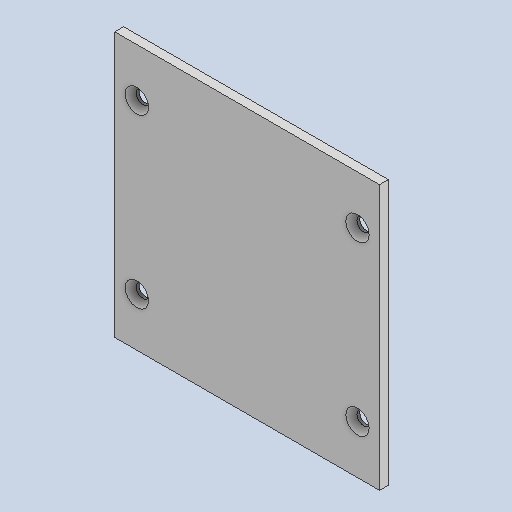
# Autodesk Inventor part: Tapa
Saved by Autodesk Inventor 2023 (Build 270158000, 158)
## iProperties
Created: 2023-04-01
Part Number: Tapa
Material: Genérico
Document SubType Name: Modeling
Designer: sergi
Density: 1 g/cm^3
Appearance: Valor por defecto
Author: sergi
Autodesk Inventor part; units mm, degrees
ref_plane "YZ Plane" through (0, 0, 0) normal (1, 0, 0) x (0, 1, 0)
ref_plane "XZ Plane" through (0, 0, 0) normal (0, 1, 0) x (-1, 0, 0)
ref_plane "XY Plane" through (0, 0, 0) normal (0, 0, 1) x (1, 0, 0)
sketch "Boceto1" plane through (0, 0, 0) normal (0, 0, 1) x (1, 0, 0)
  line L0 (-30, 30) -> (30, 30)
  line L1 (30, 30) -> (30, -30)
  line L2 (30, -30) -> (-30, -30)
  line L3 (-30, -30) -> (-30, 30)
  line L4 (-30, 30) -> (30, -30) construction
  line L5 (30, 30) -> (-30, -30) construction
  point P0 (0, 0)
  dimension "d0" = 60
  dimension "d1" = 60
  constraints: 12 end point, 2 midpoint, 2 parallel, 1 horizontal, 1 perpendicular
  measures "d0" distance of L1.end L2.end
  measures "d1" distance of L0.end L1.end
extrude "Extrusión1" add sketch "Boceto1" along normal blind 2
sketch "Boceto2" plane through (0, 0, 2) normal (0, 0, 1) x (1, 0, 0)
  circle A0 centre (-25, 19) radius 2.2 projected
  circle A1 centre (-25, -19) radius 2.2 projected
  circle A2 centre (25, -19) radius 2.2 projected
  circle A3 centre (25, 19) radius 2.2 projected
  point P0 (0, 0)
hole "Agujero1" at (25, 19, 2) at (-25, 19, 2) at (-25, -19, 2) at (25, -19, 2) direction (0, 0, -1) diameter 3 depth 2 countersink diameter 5.3 countersink angle 80
sketch "Boceto3" plane through (0, 0, 0) normal (0, 0, -1) x (-1, 0, 0)
  circle A0 centre (0, 0) radius 24.5 projected
  circle A1 centre (0, 0) radius 27
  circle A2 centre (0, 0) radius 24.5
  circle A3 centre (0, 0) radius 27.5 projected
  circle A4 centre (0, 0) radius 27.5 projected
  point P0 (12.49, 24.5)
  point P1 (12.49, -24.5)
  dimension "d13" = 54
  constraints: 2 centre point, 2 coincident, 1 concentric
  measures "d13" diameter of A1
extrude "Extrusión2" add sketch "Boceto3" along normal blind 2 contours A1
